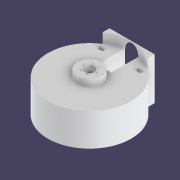
# Autodesk Inventor part: AA035c
Saved by Autodesk Inventor 2017 SP1 (Build 210196100, 196)
## iProperties
Created: 2018-03-20
Part Number: AA035c
Material: ABS Plastic
Document SubType Name: Modeling
Designer: Zach
Density: 1.06 g/cm^3
Appearance: CR White
Author: Zach
Autodesk Inventor part; units mm, degrees
ref_plane "YZ Plane" through (0, 0, 0) normal (1, 0, 0) x (0, 1, 0)
ref_plane "XZ Plane" through (0, 0, 0) normal (0, 1, 0) x (-1, 0, 0)
sketch "Sketch1" plane through (0, 0, 0) normal (0, 0, 1) x (1, 0, 0)
  circle A0 centre (0, 0) radius 60
  circle A1 centre (0, 0) radius 5
  dimension "d0" = 120
  dimension "d1" = 10
  constraints: 2 centre point, 2 coincident
  measures "d0" diameter of A0
  measures "d1" diameter of A1
extrude "Extrusion1" add sketch "Sketch1" along normal blind 67 contours A0 | A1
sketch "Sketch2" plane through (0, 0, 0) normal (0, 1, 0) x (-1, 0, 0)
  line L0 (-60, 0) -> (60, 0) projected
  line L1 (32.5, 0) -> (-32.5, 0)
  line L2 (-32.5, 0) -> (-32.5, 61)
  line L3 (-32.5, 61) -> (32.5, 61)
  line L4 (32.5, 61) -> (32.5, 0)
  point P0 (0, 0)
  point P1 (0, 0)
  dimension "d4" = 65
  dimension "d5" = 61
  constraints: 8 end point, 2 midpoint, 2 parallel, 1 horizontal, 1 perpendicular, 1 point on line
  measures "d4" distance of L2.end L3.end
  measures "d5" distance of L1.end L2.end
extrude "Extrusion2" add sketch "Sketch2" along normal blind 61.3268
sketch "Sketch3" plane through (0, 61.3268, 0) normal (0, 1, 0) x (1, 0, 0)
  line L0 (27.5, -3.5) -> (-27.5, -3.5) construction
  line L1 (-27.5, -3.5) -> (-27.5, -43.5) construction
  line L2 (-27.5, -43.5) -> (27.5, -43.5) construction
  line L3 (27.5, -43.5) -> (27.5, -3.5) construction
  line L4 (32.5, 0) -> (-32.5, 0) construction
  circle A0 centre (-27.5, -43.5) radius 2.5
  circle A1 centre (-27.5, -3.5) radius 2.5
  circle A2 centre (27.5, -3.5) radius 2.5
  circle A3 centre (27.5, -43.5) radius 2.5
  line L5 (-32.5, -61) -> (32.5, -61) projected
  point P0 (0, 0)
  point P1 (0, -3.5)
  point P2 (0, 0)
  dimension "d8" = 55
  dimension "d9" = 40
  dimension "d11" = 5
  dimension "d12" = 5
  dimension "d13" = 5
  dimension "d14" = 5
  dimension "d155" = 17.5
  constraints: 8 end point, 4 centre point, 4 coincident, 2 midpoint, 2 parallel, 1 horizontal, 1 perpendicular, 1 vertical alignment
  measures "d8" distance of L2.end L1.end
  measures "d9" distance of L1.end L0.end
  measures "d11" diameter of A0
  measures "d12" diameter of A1
  measures "d13" diameter of A2
  measures "d14" diameter of A3
  measures "d155" distance between parallel lines of L2 L5
extrude "Extrusion3" cut sketch "Sketch3" against normal blind 30
sketch "Sketch4" plane through (0, 0, 67) normal (0, 0, 1) x (1, 0, 0)
  circle A0 centre (0, 0) radius 55
  dimension "d17" = 110
  constraints: 1 centre point, 1 coincident
  measures "d17" diameter of A0
extrude "Extrusion4" cut sketch "Sketch4" against normal blind 20
sketch "Sketch5" plane through (0, 0, 47) normal (0, 0, 1) x (1, 0, 0)
  circle A0 centre (0, 0) radius 17.5
  dimension "d20" = 35
  constraints: 1 centre point, 1 coincident
  measures "d20" diameter of A0
extrude "Extrusion5" add sketch "Sketch5" along normal blind 10
sketch "Sketch6" plane through (0, 0, 57) normal (0, 0, 1) x (1, 0, 0)
  circle A0 centre (0, 0) radius 5
  dimension "d23" = 10
  constraints: 1 centre point, 1 coincident
  measures "d23" diameter of A0
extrude "Extrusion6" cut sketch "Sketch6" against normal through all
sketch "Sketch7" plane through (0, 0, 57) normal (0, 0, 1) x (1, 0, 0)
  circle A0 centre (0, 0) radius 7.5
  dimension "d26" = 15
  constraints: 1 centre point, 1 coincident
  measures "d26" diameter of A0
extrude "Extrusion7" cut sketch "Sketch7" against normal blind 5
sketch "Sketch8" plane through (0, 0, 57) normal (0, 0, 1) x (1, 0, 0)
  circle A0 centre (-9.525, 0) radius 1.5
  circle A1 centre (-4.7625, -8.2489) radius 1.5
  circle A2 centre (4.7625, -8.2489) radius 1.5
  circle A3 centre (9.525, 0) radius 1.5
  circle A4 centre (4.7625, 8.2489) radius 1.5
  circle A5 centre (-4.7625, 8.2489) radius 1.5
  point P0 (0, 0)
  dimension "d29" = 3
  dimension "d30" = 9.525
  dimension "d33" = 360
  constraints: 6 centre point, 1 horizontal alignment, 13 other
  measures "d29" diameter of A0
  measures "d30" distance of point (0, 0) A0.centre
extrude "Extrusion8" cut sketch "Sketch8" against normal blind 15
sketch "Sketch9" plane through (0, 0, 0) normal (0, 1, 0) x (-1, 0, 0)
  line L0 (-7.5, 57) -> (7.5, 57) projected
  circle A0 centre (0, 54.65) radius 1.5
  circle A1 centre (0, 59.75) radius 1.5
  line L1 (0, 59.75) -> (0, 54.65)
  line L2 (0, 58.25) -> (0, 56.15)
  point P0 (0, 0)
  point P1 (0, 57.2)
  point P2 (0, 57)
  dimension "d41" = 3
  dimension "d42" = 3
  dimension "d44" = 2.1
  dimension "d45" = 1.25
  constraints: 4 end point, 3 vertical alignment, 2 midpoint, 2 point on line, 1 vertical, 4 other
  measures "d44" distance of L2.start L2.end
  measures "d45" distance from line of L0 L2.start
extrude "Extrusion9" cut sketch "Sketch9" against normal through all
sketch "Sketch10" plane through (0, 0, 0) normal (0, 0, -1) x (-1, 0, 0)
  line L0 (0, 0) -> (-33.8074, -9.0587) construction
  line L1 (0, 0) -> (35, 0) construction
  circle A0 centre (-33.8074, -9.0587) radius 2.5
  circle A1 centre (-24.7487, 24.7487) radius 2.5
  circle A2 centre (9.0587, 33.8074) radius 2.5
  circle A3 centre (33.8074, 9.0587) radius 2.5
  circle A4 centre (24.7487, -24.7487) radius 2.5
  circle A5 centre (-9.0587, -33.8074) radius 2.5
  dimension "d48" = 35
  dimension "d49" = 165
  dimension "d50" = 5
  dimension "d53" = 360
  constraints: 6 centre point, 4 end point, 3 coincident, 1 equal length, 1 horizontal, 16 other
  measures "d48" distance of L0.start L0.end
  measures "d49" angle of L0 L1
  measures "d50" diameter of A0
extrude "Extrusion10" cut sketch "Sketch10" against normal blind 25
sketch "Sketch11" plane through (0, 0, 47) normal (0, 0, 1) x (1, 0, 0)
  line L0 (-30, 31.3268) -> (-25, 31.3268) projected
  line L1 (-30, 61.3268) -> (-25, 61.3268) projected
  line L2 (25, 31.3268) -> (30, 31.3268) projected
  line L3 (25, 61.3268) -> (30, 61.3268) projected
  line L4 (32, 41.3268) -> (23, 41.3268)
  line L5 (23, 41.3268) -> (23, 46.3268)
  line L6 (23, 46.3268) -> (32, 46.3268)
  line L7 (32, 46.3268) -> (32, 41.3268)
  line L8 (-23, 41.3268) -> (-32, 41.3268)
  line L9 (-32, 41.3268) -> (-32, 46.3268)
  line L10 (-32, 46.3268) -> (-23, 46.3268)
  line L11 (-23, 46.3268) -> (-23, 41.3268)
  point P0 (0, 0)
  point P1 (-20, 61.3268)
  point P2 (20, 61.3268)
  point P3 (25, 61.3268)
  point P4 (-27.5, 41.3268)
  point P5 (-27.5, 31.3268)
  point P6 (27.5, 41.3268)
  point P7 (27.5, 31.3268)
  dimension "d57" = 9
  dimension "d58" = 5
  dimension "d59" = 9
  dimension "d60" = 5
  dimension "d61" = 10
  constraints: 16 end point, 4 midpoint, 4 parallel, 2 horizontal, 2 perpendicular, 2 vertical alignment, 1 horizontal alignment
  measures "d57" distance of L5.end L6.end
  measures "d58" distance of L4.end L5.end
  measures "d59" distance of L9.end L10.end
  measures "d60" distance of L8.end L9.end
  measures "d61" distance between parallel lines of L2 L4
extrude "Extrusion11" cut sketch "Sketch11" against normal blind 8.5
sketch "Sketch12" plane through (0, 0, 0) normal (0, 0, -1) x (-1, 0, 0)
  line L0 (-32, 41.3268) -> (-23, 41.3268) projected
  line L1 (-32, 46.3268) -> (-32, 41.3268) projected
  line L2 (-23, 46.3268) -> (-32, 46.3268) projected
  line L3 (-23, 41.3268) -> (-23, 46.3268) projected
  line L4 (23, 41.3268) -> (32, 41.3268) projected
  line L5 (23, 46.3268) -> (23, 41.3268) projected
  line L6 (32, 46.3268) -> (23, 46.3268) projected
  line L7 (32, 41.3268) -> (32, 46.3268) projected
  point P0 (0, 0)
extrude "Extrusion12" cut sketch "Sketch12" against normal blind 8.5
sketch "Sketch14" plane through (0, 61.3268, 0) normal (0, 1, 0) x (1, 0, 0)
  circle A0 centre (0, -21) radius 10
  line L0 (32.5, 0) -> (-32.5, 0) projected
  point P0 (0, 0)
  point P1 (0, 0)
  dimension "d68" = 20
  dimension "d69" = 21
  constraints: 1 centre point, 1 midpoint, 1 vertical alignment
  measures "d68" diameter of A0
  measures "d69" distance of point (0, 0) A0.centre
extrude "Extrusion13" cut sketch "Sketch14" against normal blind 25
ref_plane "Work Plane5" through (-32.5, 61.3268, 61) normal (0, -0.8660254, 0.5) x (1, 0, 0)
sketch "Sketch30" plane through (-32.5, 61.3268, 61) normal (0, -0.8660254, 0.5) x (1, 0, 0)
  circle A0 centre (32.5, -12) radius 10
  line L0 (0, 0) -> (65, 0) projected
  point P0 (32.5, -83.491)
  point P1 (32.5, 0)
  dimension "d145" = 20
  dimension "d146" = 12
  constraints: 1 centre point, 1 midpoint, 1 vertical alignment
  measures "d145" diameter of A0
  measures "d146" distance from line of A0.centre L0
extrude "Extrusion25" cut sketch "Sketch30" along normal through all both and the other way through all
sketch "Sketch32" plane through (0, 0, 47) normal (0, 0, 1) x (1, 0, 0)
  line L0 (-10, 36.3268) -> (10, 36.3268) projected
  line L1 (-10, 61.3268) -> (10, 61.3268) projected
  line L2 (-10, 36.3268) -> (10, 36.3268) projected
  line L3 (10, 36.3268) -> (-10, 36.3268)
  line L4 (-10, 36.3268) -> (-10, 61.3268)
  line L5 (-10, 61.3268) -> (10, 61.3268)
  line L6 (10, 61.3268) -> (10, 36.3268)
  point P0 (0, 0)
  constraints: 8 end point, 2 parallel, 1 horizontal, 1 perpendicular
extrude "Extrusion27" cut sketch "Sketch32" against normal blind 26
sketch "Sketch33" plane through (0, 36.3268, 0) normal (0, 1, 0) x (1, 0, 0)
  arc A0 (10, -21) -> (-10, -21) centre (0, -21) ccw projected
  line L0 (-10, -47) -> (-10, -21) projected
  line L1 (10, -47) -> (-10, -47) projected
  line L2 (10, -47) -> (10, -21) projected
  point P0 (0, 0)
extrude "Extrusion28" cut sketch "Sketch33" against normal blind 15
sketch "Sketch34" plane through (32.5, 50.4356, 0) normal (1, 0, 0) x (0, 0, -1)
  line L0 (-67, 9.5644) -> (-67, -110.4356) projected
  line L1 (-67, -59.4356) -> (-47, -59.4356)
  line L2 (-47, -59.4356) -> (-47, -41.4356)
  line L3 (-47, -41.4356) -> (-67, -41.4356)
  line L4 (-67, -41.4356) -> (-67, -59.4356)
  line L5 (-47, 3.6477) -> (-47, -29.1088) projected
  line L6 (-47, -29.1088) -> (-47, 3.6477) projected
  line L7 (-47, -4.1088) -> (-47, 3.6477) projected
  line L8 (-47, -4.1088) -> (-47, -9.1088) projected
  line L9 (-47, -9.1088) -> (-47, -5.7031) projected
  line L10 (-47, -5.7031) -> (-47, -5.7031) projected
  line L11 (-47, -5.7031) -> (-47, -9.1088) projected
  line L12 (-47, -9.1088) -> (-47, -4.1088) projected
  line L13 (-47, 3.6477) -> (-47, -4.1088) projected
  line L14 (-47, -67.9356) -> (-47, -32.9356) projected
  line L15 (-47, -59.4356) -> (-67, -79.4356)
  line L16 (-67, -105.4356) -> (-67, 4.5644) projected
  line L17 (-47, -41.4356) -> (-67, -21.4356)
  line L18 (-67, -79.4356) -> (-67, -59.4356)
  line L19 (-67, -21.4356) -> (-67, -41.4356)
  point P0 (0, -50.4356)
  point P1 (-67, -50.4356)
  dimension "d160" = 18
  dimension "d163" = 20
  dimension "d164" = 45
  dimension "d165" = 45
  constraints: 16 end point, 3 point on line, 2 collinear, 2 midpoint, 2 parallel, 1 horizontal, 1 perpendicular
  measures "d160" distance between parallel lines of L3 L1
  measures "d163" distance between parallel lines of L0 L2
  measures "d164" angle of L15 L1
  measures "d165" angle of L3 L17
extrude "Extrusion29" cut sketch "Sketch34" along normal through all
fillet "Fillet2" radius 20 2 edges at (49.6297, 29, 67) (49.6297, -29, 67)
fillet "Fillet3" radius 5 2 edges at (56.7899, -9, 47) (56.7899, 9, 47)
fillet "Fillet5" radius 2 9 edges at (46.054, 30.067, 65.6524) (52.3301, 16.928, 54.928) (54.2687, 8.9389, 47.4218) (54.4201, -7.9659, 47) (54.4201, 7.9659, 47) (54.2687, -8.9389, 47.4218) (52.3301, -16.928, 54.928) (46.054, -30.067, 65.6524) (-55, 0, 67)
sketch "Sketch35" plane through (0, 0, 47) normal (0, 0, 1) x (1, 0, 0)
  circle A0 centre (0, 0) radius 17.5 projected
  arc A1 (47.0094, 37.2843) -> (47.0094, -37.2843) centre (0, 0) ccw construction
  circle A2 centre (0, 0) radius 60 construction
  circle A3 centre (0, 0) radius 61
  dimension "d171" = 1
  constraints: 1 centre point, 1 coincident, 3 other
extrude "Extrusion30" cut sketch "Sketch35" along normal through all
equation "\"d24\" = d23"
body "Solid1"
